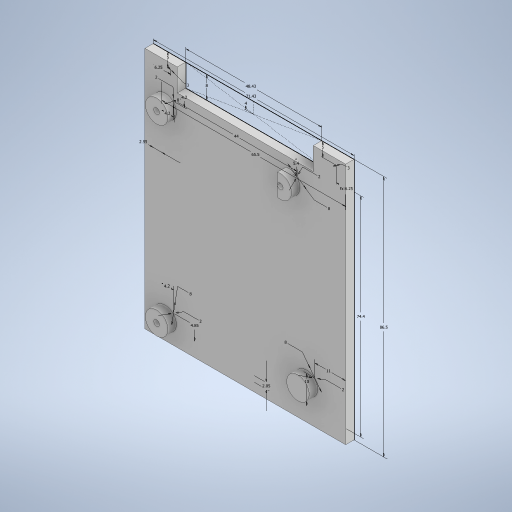
# Autodesk Inventor part: Component_shield_layered_PCB_platform
Saved by Autodesk Inventor 2024 (Build 280153000, 153)
## iProperties
Created: 2024-10-22
Part Number: Component_shield_layered_PCB_platform
Material: Generic
Document SubType Name: Modeling
Designer: Bruger
Density: 1 g/cm^3
Appearance: Default
Author: Bruger
Autodesk Inventor part; units mm, degrees
ref_plane "YZ Plane" through (0, 0, 0) normal (1, 0, 0) x (0, 1, 0)
ref_plane "XZ Plane" through (0, 0, 0) normal (0, 1, 0) x (-1, 0, 0)
ref_plane "XY Plane" through (0, 0, 0) normal (0, 0, 1) x (1, 0, 0)
sketch "Sketch1" plane through (0, 0, 0) normal (0, 0, 1) x (1, 0, 0)
  line L0 (0, 0) -> (71.43, 0)
  line L1 (71.43, 0) -> (71.43, 86.5)
  line L2 (71.43, 86.5) -> (0, 86.5)
  line L3 (0, 86.5) -> (0, 0)
  line L4 (14, 86.5) -> (57.43, 86.5)
  circle A0 centre (6.25, 81.5) radius 1.5
  circle A1 centre (65.18, 81.5) radius 1.5
  line L5 (11.5, 78.5) -> (59.93, 78.5)
  line L6 (59.93, 78.5) -> (59.93, 86.5)
  line L7 (59.93, 86.5) -> (11.5, 86.5)
  line L8 (11.5, 86.5) -> (11.5, 78.5)
  line L9 (11.5, 78.5) -> (59.93, 86.5) construction
  line L10 (59.93, 78.5) -> (11.5, 86.5) construction
  line L11 (35.715, 86.5) -> (35.715, 82.5) construction
  line L12 (2.95, 2.05) -> (68.45, 2.05)
  line L13 (68.45, 2.05) -> (68.45, 76.45)
  line L14 (68.45, 76.45) -> (2.95, 76.45)
  line L15 (2.95, 76.45) -> (2.95, 2.05)
  line L16 (2.95, 2.05) -> (68.45, 76.45) construction
  line L17 (68.45, 2.05) -> (2.95, 76.45) construction
  circle A2 centre (7.15, 72.25) radius 4
  circle A3 centre (51.15, 71.05) radius 4
  circle A4 centre (7.15, 6.9) radius 4
  circle A5 centre (57.45, 12.05) radius 4
  circle A6 centre (7.15, 72.25) radius 1
  circle A7 centre (51.15, 71.05) radius 1
  circle A8 centre (7.15, 6.9) radius 1
  circle A9 centre (57.45, 12.05) radius 1
  line L18 (50.15, 74.923) -> (50.15, 67.177)
  point P0 (11.5, 86.5)
  point P1 (35.7, 39.25)
  point P2 (35.715, 0)
  point P3 (35.7, 2.05)
  point P4 (9.1397, 10.37)
  point P5 (9.1397, 3.43)
  point P6 (8.15, 10.773)
  point P7 (8.15, 3.027)
  dimension "d0" = 71.43
  dimension "d1" = 86.5
  dimension "d8" = 3
  dimension "d9" = 6.25
  dimension "d10" = 5
  dimension "d11" = 3
  dimension "d12" = 5
  dimension "d13" = 6.25
  dimension "d15" = 48.43
  dimension "d16" = 8
  dimension "d17" = 4
  dimension "d19" = 65.5
  dimension "d20" = 74.4
  dimension "d21" = 2.05
  dimension "d22" = 2.95
  dimension "d23" = 4.2
  dimension "d24" = 4.2
  dimension "d25" = 8
  dimension "d26" = 8
  dimension "d27" = 5.4
  dimension "d29" = 4.85
  dimension "d30" = 4.2
  dimension "d31" = 8
  dimension "d34" = 8
  dimension "d35" = 11
  dimension "d36" = 10
  dimension "d37" = 2
  dimension "d38" = 2
  dimension "d39" = 2
  dimension "d40" = 2
  dimension "d55" = 44
  constraints: 38 end point, 10 centre point, 7 midpoint, 6 parallel, 6 point on circle, 4 coincident, 4 horizontal, 4 perpendicular, 1 point on line, 1 vertical
  measures "d0" distance of L1.end L2.end
  measures "d1" distance between parallel lines of L0 L2
  measures "d8" diameter of A0
  measures "d9" distance from line of L3 A0.centre
  measures "d10" distance from line of L2 A0.centre
  measures "d11" diameter of A1
  measures "d12" distance from line of L2 A1.centre
  measures "d13" distance from line of A1.centre L1
  measures "d15" distance of L7.end L6.end
  measures "d16" distance between parallel lines of L4 L5
  measures "d17" distance of L11.start L11.end
  measures "d19" distance of L14.end L13.end
  measures "d20" distance of L13.end L12.end
  measures "d21" vertical distance of point (35.715, 0) point (35.7, 2.05)
  measures "d22" distance between parallel lines of L3 L15
  measures "d23" distance from line of L14 A2.centre
  measures "d24" distance from line of A2.centre L15
  measures "d25" diameter of A2
  measures "d26" diameter of A3
  measures "d27" distance from line of L14 A3.centre
  measures "d29" distance from line of A4.centre L12
  measures "d30" distance from line of A4.centre L15
  measures "d31" diameter of A4
  measures "d34" diameter of A5
  measures "d35" distance from line of L13 A5.centre
  measures "d36" distance from line of L12 A5.centre
  measures "d37" diameter of A6
  measures "d38" diameter of A7
  measures "d39" diameter of A8
  measures "d40" diameter of A9
  measures "d55" horizontal distance of A2.centre A3.centre
extrude "Extrusion1" add sketch "Sketch1" along normal blind 3 contours L3 L2 L8 L5 L6 L1 L0 | A0 | A1 | L15 L14 L13 L12 | A2 | A7 | A3 L18 | L18 A3 | A4 | A5 | A6 | A8 | A9
extrude "Extrusion2" add sketch "Sketch1" along normal blind 6 contours A2 | A7 | A3 L18 | A4 | A5 | A6 | A8 | A9 picked at (54.1155, 70.7487)
hole "Hole2" at (51.15, 71.05, 0) at (7.15, 72.25, 0) at (7.15, 6.9, 0) direction (0, 0, 1) diameter 2 end through all
equation "\"d13\" = d9"
body "Solid1"
